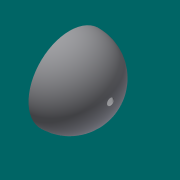
# Autodesk Inventor part: MuzzleEnd
Saved by Autodesk Inventor 2020.4 (Build 244396010, 396A)
## iProperties
Created: 2022-09-11
Part Number: MuzzleEnd
Material: Generic
Document SubType Name: Modeling
Designer: Val
Density: 1 g/cm^3
Appearance: Default
Author: Val
Autodesk Inventor part; units mm, degrees
ref_plane "YZ Plane" through (0, 0, 0) normal (1, 0, 0) x (0, 1, 0)
ref_plane "XZ Plane" through (0, 0, 0) normal (0, 1, 0) x (-1, 0, 0)
ref_plane "XY Plane" through (0, 0, 0) normal (0, 0, 1) x (1, 0, 0)
sketch "Profile" plane through (0, 0, 0) normal (0, 0, 1) x (1, 0, 0)
  line L0 (0, 0) -> (95.25, 0) construction
  arc A0 (19.05, 0) -> (95.25, -76.2) centre (95.25, 0) ccw construction
  line L1 (95.25, 76.2) -> (0, 76.2) construction
  line L2 (0, -76.2) -> (95.25, -76.2) construction
  line L3 (95.25, -76.2) -> (95.25, 76.2) construction
  arc A1 (95.25, 76.2) -> (19.05, 0) centre (95.25, 0) ccw construction
  arc A2 (95.25, -76.2) -> (171.45, 0) centre (95.25, 0) ccw construction
  line L4 (95.25, 0) -> (171.45, 0) construction
  arc A3 (171.45, 0) -> (95.25, 76.2) centre (95.25, 0) ccw
  line L5 (0, 0) -> (0, -76.2) construction
  line L6 (0, 0) -> (171.45, 0)
  arc A4 (169.45, 0) -> (95.25, 74.2) centre (95.25, 0) ccw
  line L7 (0, 76.2) -> (0, 74.2) construction
  line L8 (0, 74.2) -> (95.25, 74.2) construction
  line L9 (95.25, 74.2) -> (95.25, 76.2)
  dimension "d0" = 76.2
  dimension "d1" = 95.25
  dimension "d4" = 2
  dimension "d8" = 95.25
  dimension "d9" = 152.4
  constraints: 20 end point, 10 point on circle, 5 centre point, 4 horizontal, 2 parallel, 2 point on line, 2 vertical, 1 coincident, 1 midpoint, 1 perpendicular, 1 tangent
  measures "d0" radius of A2
  measures "d1" distance of L1.start L1.end
  measures "d4" distance of L1.end L7.end
  measures "d8" distance between parallel lines of L5 L3
  measures "d9" distance of L2.end L1.start
revolve "ProfileFeature" add sketch "Profile" angle 360 about axis through (0, 0, 0) along (1, 0, 0)
sketch "CenterHole" plane through (95.25, 0, 0) normal (-1, 0, 0) x (0, 0, 1)
  circle A0 centre (0, 0) radius 6.35
  dimension "d5" = 12.7
  constraints: 1 centre point, 1 coincident
  measures "d5" diameter of A0
extrude "CenterHoleFeature" cut sketch "CenterHole" against normal through all
body "Solid1"
